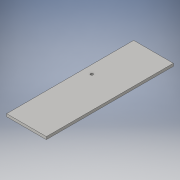
# Autodesk Inventor part: baseForWormMotor
Saved by Autodesk Inventor 2016 (Build 200138000, 138)
## iProperties
Created: 2015-06-16
Part Number: baseForWormMotor
Material: Generic
Document SubType Name: Modeling
Designer: steele
Density: 1 g/cm^3
Appearance: Default
Author: steele
Autodesk Inventor part; units mm, degrees
ref_plane "YZ Plane" through (0, 0, 0) normal (1, 0, 0) x (0, 1, 0)
ref_plane "XZ Plane" through (0, 0, 0) normal (0, 1, 0) x (-1, 0, 0)
ref_plane "XY Plane" through (0, 0, 0) normal (0, 0, 1) x (1, 0, 0)
sketch "Sketch1" plane through (0, 0, 0) normal (0, 1, 0) x (-1, 0, 0)
  line L0 (-47.625, 152.4) -> (-47.625, -152.4)
  line L1 (-47.625, -152.4) -> (47.625, -152.4)
  line L2 (47.625, -152.4) -> (47.625, 152.4)
  line L3 (47.625, 152.4) -> (-47.625, 152.4)
  line L4 (-47.625, 152.4) -> (47.625, -152.4) construction
  line L5 (-47.625, -152.4) -> (47.625, 152.4) construction
  point P0 (0, 0)
  dimension "d0" = 304.8
  dimension "d1" = 95.25
  constraints: 12 end point, 2 midpoint, 2 parallel, 1 perpendicular, 1 vertical
  measures "d0" distance of L0.start L0.end
  measures "d1" distance of L1.end L0.end
extrude "Extrusion1" add sketch "Sketch1" along normal blind 6.35
sketch "Sketch3" plane through (0, 6.35, 0) normal (0, 1, 0) x (1, 0, 0)
  line L0 (-47.5869, 31.75) -> (47.625, 31.75) construction
  line L1 (47.625, -152.4) -> (47.625, 152.4) construction
  line L2 (-27.5209, 152.4) -> (-27.5209, -152.4) construction
  line L3 (47.625, 152.4) -> (-47.625, 152.4) projected
  circle A0 centre (-27.5209, 31.75) radius 3.175
  point P0 (0, 0)
  dimension "d9" = 27.5209
  dimension "d10" = 120.65
  dimension "d11" = 6.35
  constraints: 4 end point, 3 point on line, 1 centre point, 1 horizontal, 1 vertical
  measures "d9" distance from line of point (0, 0) L2
  measures "d10" distance between parallel lines of L3 L0
  measures "d11" diameter of A0
extrude "Extrusion3" cut sketch "Sketch3" against normal through all
body "Solid1"
